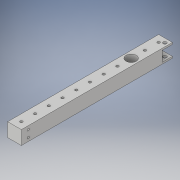
# Autodesk Inventor part: RobotArm Arm2
Saved by Autodesk Inventor 2018 (Build 220112000, 112)
## iProperties
Created: 2018-01-20
Part Number: RobotArm Arm2
Material: Generic
Document SubType Name: Modeling
Designer: lopez.xavier
Density: 1 g/cm^3
Appearance: Default
Author: lopez.xavier
Autodesk Inventor part; units mm, degrees
ref_plane "YZ Plane" through (0, 0, 0) normal (1, 0, 0) x (0, 1, 0)
ref_plane "XZ Plane" through (0, 0, 0) normal (0, 1, 0) x (-1, 0, 0)
ref_plane "XY Plane" through (0, 0, 0) normal (0, 0, 1) x (1, 0, 0)
sketch "Sketch1" plane through (0, 0, 0) normal (0, 0, 1) x (1, 0, 0)
  line L0 (0, 0) -> (25.4, 0)
  line L1 (25.4, 0) -> (25.4, 25.4)
  line L2 (25.4, 25.4) -> (0, 25.4)
  line L3 (0, 25.4) -> (0, 0)
  dimension "d0" = 25.4
  dimension "d1" = 25.4
  constraints: 8 end point, 2 parallel, 1 horizontal, 1 perpendicular
  measures "d0" distance of L1.end L2.end
  measures "d1" distance of L0.end L1.end
extrude "Extrusion1" add sketch "Sketch1" along normal blind 279.4
sketch "Sketch2" plane through (0, 25.4, 0) normal (0, 1, 0) x (1, 0, 0)
  circle A0 centre (12.7, -12.7) radius 2.3813
  line L0 (25.4, 0) -> (0, 0) projected
  line L1 (0, 0) -> (0, -279.4) projected
  circle A1 centre (12.7, -38.1) radius 2.3813
  circle A2 centre (12.7, -63.5) radius 2.3813
  circle A3 centre (12.7, -88.9) radius 2.3813
  circle A4 centre (12.7, -114.3) radius 2.3813
  circle A5 centre (12.7, -139.7) radius 2.3813
  circle A6 centre (12.7, -165.1) radius 2.3813
  circle A7 centre (12.7, -190.5) radius 2.3813
  circle A8 centre (12.7, -215.9) radius 2.3813
  circle A9 centre (12.7, -241.3) radius 2.3813
  circle A10 centre (12.7, -266.7) radius 2.3813
  circle A11 centre (12.7, -63.5) radius 9.525
  circle A12 centre (19.05, -7.62) radius 3.175
  line L2 (25.4, 0) -> (25.4, -279.4) projected
  dimension "d4" = 4.7625
  dimension "d5" = 12.7
  dimension "d6" = 12.7
  dimension "d9" = 25.4
  dimension "d14" = 19.05
  dimension "d25" = 6.35
  dimension "d27" = 6.35
  dimension "d28" = 55.88
  constraints: 13 centre point, 1 coincident, 1 vertical, 20 other
  measures "d4" diameter of A0
  measures "d5" distance from line of L0 A0.centre
  measures "d6" distance from line of L1 A0.centre
  measures "d9" distance of A0.centre A1.centre
  measures "d14" diameter of A11
  measures "d25" diameter of A12
  measures "d27" distance from line of L2 A12.centre
  measures "d28" vertical distance of A11.centre A12.centre
extrude "Extrusion2" cut sketch "Sketch2" against normal blind 279.4 contours A0 | A1 | A2 | A3 | A4 | A5 | A6 | A7 | A8 | A9 | A10 | A11 | A12
sketch "Sketch3" plane through (25.4, 0, 0) normal (1, 0, 0) x (0, 0, -1)
  line L0 (-19.05, 22.225) -> (0, 22.225)
  line L1 (0, 22.225) -> (0, 3.175)
  line L2 (0, 3.175) -> (-19.05, 3.175)
  line L3 (-19.05, 3.175) -> (-19.05, 22.225)
  line L4 (0, 0) -> (0, 25.4) projected
  line L5 (0, 0) -> (-279.4, 0) projected
  line L6 (0, 25.4) -> (-279.4, 25.4) projected
  dimension "d17" = 0
  dimension "d18" = 19.05
  dimension "d19" = 3.175
  dimension "d20" = 3.175
  constraints: 8 end point, 2 parallel, 1 horizontal, 1 perpendicular
  measures "d17" distance between parallel lines of L4 L1
  measures "d18" distance of L0.start L0.end
  measures "d19" distance between parallel lines of L5 L2
  measures "d20" distance between parallel lines of L6 L0
extrude "Extrusion3" cut sketch "Sketch3" against normal blind 279.4
sketch "Sketch4" plane through (25.4, 0, 279.4) normal (1, 0, 0) x (0, 0, -1)
  circle A0 centre (12.7, 6.2992) radius 2.0701
  line L0 (0, 0) -> (0, 25.4) projected
  circle A1 centre (12.7, 18.9992) radius 2.0701
  line L1 (279.4, 0) -> (0, 0) projected
  line L2 (279.4, 25.4) -> (0, 25.4) projected
  dimension "d29" = 4.1402
  dimension "d30" = 12.7
  dimension "d31" = 4.1402
  dimension "d32" = 12.7
  dimension "d34" = 12.7
  dimension "d37" = 6.4008
  constraints: 2 centre point
  measures "d29" diameter of A0
  measures "d30" distance from line of L0 A0.centre
  measures "d31" diameter of A1
  measures "d32" distance from line of L0 A1.centre
  measures "d34" distance of A0.centre A1.centre
  measures "d37" distance from line of L2 A1.centre
extrude "Extrusion4" cut sketch "Sketch4" against normal blind 25.4
equation "\"d20\" = d19"
equation "\"d31\" = d29"
equation "\"d32\" = d30"
body "Solid1"
